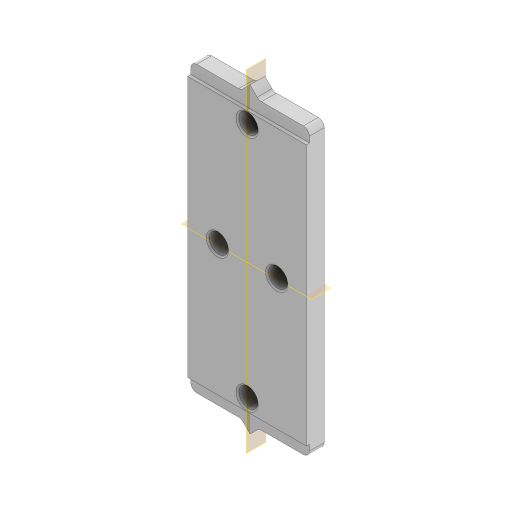
# Autodesk Inventor part: Klemmplatte
Saved by Autodesk Inventor 2024.3 (Build 283343000, 343)
## iProperties
Created: 2025-05-14
Part Number: Klemmplatte
Material: Generisch
Document SubType Name: Modeling
Designer: Demir
Density: 1 g/cm^3
Appearance: Vorgabe
Author: Demir
Autodesk Inventor part; units mm, degrees
ref_plane "XZ Plane" through (0, 0, 0) normal (0, 1, 0) x (-1, 0, 0)
sketch "Skizze1" plane through (0, 0, 0) normal (0, 0, 1) x (1, 0, 0)
  line L0 (-20, 3) -> (20, 3)
  line L1 (20, 3) -> (20, -3)
  line L2 (20, -3) -> (-20, -3)
  line L3 (-20, -3) -> (-20, 3)
  line L4 (-20, 3) -> (20, -3) construction
  line L5 (20, 3) -> (-20, -3) construction
  point P0 (0, 0)
  dimension "d0" = 6
  dimension "d2" = 40
  constraints: 12 end point, 2 midpoint, 2 parallel, 1 horizontal, 1 perpendicular
  measures "d0" distance of L0.end L1.end
  measures "d2" distance of L1.end L2.end
extrude "Extrusion1" add sketch "Skizze1" along normal mid plane 96
sketch "Skizze3" plane through (-20, 3, 48) normal (0, 1, 0) x (1, 0, 0)
  line L0 (0, 96) -> (0, 0) projected
  line L1 (40, 0) -> (0, 0) projected
  line L2 (40, 96) -> (40, 0) projected
  line L3 (0, 96) -> (40, 96) projected
  point P0 (20, 48)
  point P1 (10, 48)
  point P2 (30, 48)
  point P3 (0, 48)
  dimension "d5" = 10
  dimension "d6" = 10
  constraints: 2 horizontal alignment, 1 midpoint
  measures "d5" distance of point (10, 48) point (0, 48)
  measures "d6" distance from line of point (30, 48) L2
hole "Bohrung1" at (-10, 3, 0) at (10, 3, 0) direction (0, -1, 0) diameter 6.5 end through all
sketch "Skizze4" plane through (-20, 3, 48) normal (0, 1, 0) x (1, 0, 0)
  circle A0 centre (30, 48) radius 3.25 projected
  circle A1 centre (10, 48) radius 3.25 projected
  line L0 (0, 96) -> (0, 0) projected
  line L1 (40, 0) -> (0, 0) projected
  line L2 (40, 96) -> (40, 0) projected
  line L3 (0, 96) -> (40, 96) projected
  point P0 (20, 48)
  point P1 (20, 8)
  point P2 (20, 88)
  dimension "d14" = 40
  dimension "d15" = 40
  constraints: 2 vertical alignment
  measures "d14" distance of point (20, 48) point (20, 8)
  measures "d15" distance of point (20, 88) point (20, 48)
hole "Bohrung2" at (0, 3, 40) at (0, 3, -40) direction (0, -1, 0) diameter 6.5 end through all
sketch "Skizze5" plane through (-20, 3, 48) normal (0, 1, 0) x (1, 0, 0)
  circle A0 centre (20, 88) radius 3.25 projected
  circle A1 centre (20, 8) radius 3.25 projected
  circle A2 centre (30, 48) radius 3.25 projected
  circle A3 centre (10, 48) radius 3.25 projected
  line L0 (0, 96) -> (0, 0) projected
  line L1 (40, 0) -> (0, 0) projected
  line L2 (40, 96) -> (40, 0) projected
  line L3 (0, 96) -> (40, 96) projected
  line L4 (20, 115.8) -> (20, -22.8) projected
  line L5 (40, 0) -> (0, 0) projected
  line L6 (20, -3) -> (23, 0)
  line L7 (20, -3) -> (17, 0)
  line L8 (0, 0) -> (40, 0) projected
  point P0 (20, 48)
  dimension "d29" = 6
  dimension "d30" = 3
  dimension "d31" = 45
  constraints: 4 end point, 3 point on line
  measures "d29" distance of L7.end L6.end
  measures "d30" horizontal distance of A1.centre L7.end
  measures "d31" angle of L6 L1
extrude "Extrusion2" add sketch "Skizze5" against normal up to surface (6 mm away) contours L4 L7 L1 | L1 L6 L4
mirror "Spiegeln1" about plane through (0, 0, 0) normal (1, 0, 0) of "Extrusion2"
mirror "Spiegeln2" about plane through (0, 0, 0) normal (0, 0, 1) of "Extrusion2", "Spiegeln1"
fillet "Rundung1" radius 2 4 edges at (-20, 0, 48) (20, 0, 48) (-20, 0, -48) (20, 0, -48)
fillet "Rundung2" radius 2 4 edges at (-3, 0, 48) (3, 0, 48) (-3, 0, -48) (3, 0, -48)
sketch "Skizze6" plane through (20, -3, -46) normal (0, -1, 0) x (1, 0, 0)
  circle A0 centre (-20, 6) radius 3.25 projected
  circle A1 centre (-20, 86) radius 3.25 projected
  circle A2 centre (-10, 46) radius 3.25 projected
  circle A3 centre (-30, 46) radius 3.25 projected
  arc A4 (-2, -2) -> (0, 0) centre (-2, 0) ccw projected
  line L0 (0, 0) -> (0, 92) projected
  arc A5 (0, 92) -> (-2, 94) centre (-2, 92) ccw projected
  line L1 (-16.1716, 94) -> (-2, 94) projected
  arc A6 (-17.5858, 94.5858) -> (-16.1716, 94) centre (-16.1716, 96) ccw projected
  line L2 (-20, 97) -> (-17.5858, 94.5858) projected
  line L3 (-22.4142, 94.5858) -> (-20, 97) projected
  arc A7 (-23.8284, 94) -> (-22.4142, 94.5858) centre (-23.8284, 96) ccw projected
  line L4 (-38, 94) -> (-23.8284, 94) projected
  arc A8 (-38, 94) -> (-40, 92) centre (-38, 92) ccw projected
  line L5 (-40, 92) -> (-40, 0) projected
  arc A9 (-40, 0) -> (-38, -2) centre (-38, 0) ccw projected
  line L6 (-23.8284, -2) -> (-38, -2) projected
  arc A10 (-22.4142, -2.5858) -> (-23.8284, -2) centre (-23.8284, -4) ccw projected
  line L7 (-22.4142, -2.5858) -> (-20, -5) projected
  line L8 (-20, -5) -> (-17.5858, -2.5858) projected
  arc A11 (-16.1716, -2) -> (-17.5858, -2.5858) centre (-16.1716, -4) ccw projected
  line L9 (-2, -2) -> (-16.1716, -2) projected
  line L10 (-59.3165, 111.9132) -> (18.0456, 111.9132)
  line L11 (18.0456, 111.9132) -> (18.0456, 90)
  line L12 (18.0456, 90) -> (-59.3165, 90)
  line L13 (-59.3165, 90) -> (-59.3165, 111.9132)
  line L14 (-80.9876, 2) -> (21.6776, 2)
  line L15 (21.6776, 2) -> (21.6776, -24.7559)
  line L16 (21.6776, -24.7559) -> (-80.9876, -24.7559)
  line L17 (-80.9876, -24.7559) -> (-80.9876, 2)
  point P0 (-20, 46)
  point P1 (-40, 2)
  point P2 (0, 2)
  dimension "d34" = 4
  dimension "d35" = 4
  dimension "d36" = 77.3621
  dimension "d37" = 21.9132
  dimension "d38" = 102.6652
  dimension "d39" = 26.7559
  constraints: 16 end point, 4 parallel, 2 horizontal, 2 perpendicular
  measures "d34" distance from line of A0.centre L14
  measures "d35" distance from line of A1.centre L12
  measures "d36" distance of L10.start L10.end
  measures "d37" distance of L10.end L11.end
  measures "d38" distance of L15.end L16.end
  measures "d39" distance of L14.end L15.end
extrude "Extrusion3" cut sketch "Skizze6" against normal blind 1 contours L9 A11 L8 L7 A10 L6 A9 L5 L14 L0 A4 | A4 L0 L14 L15 L16 L17 L5 A9 L6 A10 L7 L8 A11 L9 | L12 L5 A8 L4 A7 L3 L2 A6 L1 A5 L0 | L0 A5 L1 A6 L2 L3 A7 L4 A8 L5 L12 L13 L10 L11
chamfer "Fasen1" distance 0.5 angle 45 4 edges at (-10, -3, -3.25) (-10, 3, -3.25) (10, -3, -3.25) (10, 3, -3.25)
chamfer "Fasen2" distance 0.5 angle 45 2 edges at (0, -3, 36.75) (0, 3, 36.75)
chamfer "Fasen3" distance 0.5 angle 45 2 edges at (0, -3, -43.25) (0, 3, -43.25)
